Autodesk Fusion 360 part; units mm, degrees
(part 5 of 10)
  line L467 (-6.3, 22.99) -> (-5.3, 22.99)
  line L468 (-5.3, 20.36) -> (-5.3, 19.36)
  line L469 (-5.3, 19.36) -> (-6.3, 19.36)
  line L470 (-6.3, 19.36) -> (-6.3, 20.36)
  line L471 (-6.3, 20.36) -> (-5.3, 20.36)
  line L472 (-5.3, 17.73) -> (-5.3, 16.73)
  line L473 (-5.3, 16.73) -> (-6.3, 16.73)
  line L474 (-6.3, 16.73) -> (-6.3, 17.73)
  line L475 (-6.3, 17.73) -> (-5.3, 17.73)
  line L476 (-5.3, 15.1) -> (-5.3, 14.1)
  line L477 (-5.3, 14.1) -> (-6.3, 14.1)
  line L478 (-6.3, 14.1) -> (-6.3, 15.1)
  line L479 (-6.3, 15.1) -> (-5.3, 15.1)
  line L480 (-5.3, 12.47) -> (-5.3, 11.47)
  line L481 (-5.3, 11.47) -> (-6.3, 11.47)
  line L482 (-6.3, 11.47) -> (-6.3, 12.47)
  line L483 (-6.3, 12.47) -> (-5.3, 12.47)
  line L484 (-5.3, 9.84) -> (-5.3, 8.84)
  line L485 (-5.3, 8.84) -> (-6.3, 8.84)
  line L486 (-6.3, 8.84) -> (-6.3, 9.84)
  line L487 (-6.3, 9.84) -> (-5.3, 9.84)
  line L488 (-5.3, 7.21) -> (-5.3, 6.21)
  line L489 (-5.3, 6.21) -> (-6.3, 6.21)
  line L490 (-6.3, 6.21) -> (-6.3, 7.21)
  line L491 (-6.3, 7.21) -> (-5.3, 7.21)
  line L492 (-5.3, 4.58) -> (-5.3, 3.58)
  line L493 (-5.3, 3.58) -> (-6.3, 3.58)
  line L494 (-6.3, 3.58) -> (-6.3, 4.58)
  line L495 (-6.3, 4.58) -> (-5.3, 4.58)
  line L496 (-5.3, 1.95) -> (-5.3, 0.95)
  line L497 (-5.3, 0.95) -> (-6.3, 0.95)
  line L498 (-6.3, 0.95) -> (-6.3, 1.95)
  line L499 (-6.3, 1.95) -> (-5.3, 1.95)
  line L500 (-5.3, -0.68) -> (-5.3, -1.68)
  line L501 (-5.3, -1.68) -> (-6.3, -1.68)
  line L502 (-6.3, -1.68) -> (-6.3, -0.68)
  line L503 (-6.3, -0.68) -> (-5.3, -0.68)
  line L504 (-5.3, -3.31) -> (-5.3, -4.31)
  line L505 (-5.3, -4.31) -> (-6.3, -4.31)
  line L506 (-6.3, -4.31) -> (-6.3, -3.31)
  line L507 (-6.3, -3.31) -> (-5.3, -3.31)
  line L508 (-5.3, -5.94) -> (-5.3, -6.94)
  line L509 (-5.3, -6.94) -> (-6.3, -6.94)
  line L510 (-6.3, -6.94) -> (-6.3, -5.94)
  line L511 (-6.3, -5.94) -> (-5.3, -5.94)
  line L512 (-5.3, -8.57) -> (-5.3, -9.57)
  line L513 (-5.3, -9.57) -> (-6.3, -9.57)
  line L514 (-6.3, -9.57) -> (-6.3, -8.57)
  line L515 (-6.3, -8.57) -> (-5.3, -8.57)
  line L516 (-5.3, -11.2) -> (-5.3, -12.2)
  line L517 (-5.3, -12.2) -> (-6.3, -12.2)
  line L518 (-6.3, -12.2) -> (-6.3, -11.2)
  line L519 (-6.3, -11.2) -> (-5.3, -11.2)
  line L520 (-5.3, -13.83) -> (-5.3, -14.83)
  line L521 (-5.3, -14.83) -> (-6.3, -14.83)
  line L522 (-6.3, -14.83) -> (-6.3, -13.83)
  line L523 (-6.3, -13.83) -> (-5.3, -13.83)
  line L524 (-5.3, -16.46) -> (-5.3, -17.46)
  line L525 (-5.3, -17.46) -> (-6.3, -17.46)
  line L526 (-6.3, -17.46) -> (-6.3, -16.46)
  line L527 (-6.3, -16.46) -> (-5.3, -16.46)
  line L528 (-5.3, -19.09) -> (-5.3, -20.09)
  line L529 (-5.3, -20.09) -> (-6.3, -20.09)
  line L530 (-6.3, -20.09) -> (-6.3, -19.09)
  line L531 (-6.3, -19.09) -> (-5.3, -19.09)
  line L532 (-5.3, -21.72) -> (-5.3, -22.72)
  line L533 (-5.3, -22.72) -> (-6.3, -22.72)
  line L534 (-6.3, -22.72) -> (-6.3, -21.72)
  line L535 (-6.3, -21.72) -> (-5.3, -21.72)
  line L536 (-5.3, -24.35) -> (-5.3, -25.35)
  line L537 (-5.3, -25.35) -> (-6.3, -25.35)
  line L538 (-6.3, -25.35) -> (-6.3, -24.35)
  line L539 (-6.3, -24.35) -> (-5.3, -24.35)
  line L540 (-5.3, -26.98) -> (-5.3, -27.98)
  line L541 (-5.3, -27.98) -> (-6.3, -27.98)
  line L542 (-6.3, -27.98) -> (-6.3, -26.98)
  line L543 (-6.3, -26.98) -> (-5.3, -26.98)
  line L544 (-5.3, -29.61) -> (-5.3, -30.61)
  line L545 (-5.3, -30.61) -> (-6.3, -30.61)
  line L546 (-6.3, -30.61) -> (-6.3, -29.61)
  line L547 (-6.3, -29.61) -> (-5.3, -29.61)
  line L548 (-5.3, -32.24) -> (-5.3, -33.24)
  line L549 (-5.3, -33.24) -> (-6.3, -33.24)
  line L550 (-6.3, -33.24) -> (-6.3, -32.24)
  line L551 (-6.3, -32.24) -> (-5.3, -32.24)
  line L552 (-5.3, -34.87) -> (-5.3, -35.87)
  line L553 (-5.3, -35.87) -> (-6.3, -35.87)
  line L554 (-6.3, -35.87) -> (-6.3, -34.87)
  line L555 (-6.3, -34.87) -> (-5.3, -34.87)
  line L556 (-5.3, -37.5) -> (-5.3, -38.5)
  line L557 (-5.3, -38.5) -> (-6.3, -38.5)
  line L558 (-6.3, -38.5) -> (-6.3, -37.5)
  line L559 (-6.3, -37.5) -> (-5.3, -37.5)
  line L560 (-2.5, 38.77) -> (-2.5, 37.77)
  line L561 (-2.5, 37.77) -> (-3.5, 37.77)
  line L562 (-3.5, 37.77) -> (-3.5, 38.77)
  line L563 (-3.5, 38.77) -> (-2.5, 38.77)
  line L564 (-2.5, 36.14) -> (-2.5, 35.14)
  line L565 (-2.5, 35.14) -> (-3.5, 35.14)
  line L566 (-3.5, 35.14) -> (-3.5, 36.14)
  line L567 (-3.5, 36.14) -> (-2.5, 36.14)
  line L568 (-2.5, 33.51) -> (-2.5, 32.51)
  line L569 (-2.5, 32.51) -> (-3.5, 32.51)
  line L570 (-3.5, 32.51) -> (-3.5, 33.51)
  line L571 (-3.5, 33.51) -> (-2.5, 33.51)
  line L572 (-2.5, 30.88) -> (-2.5, 29.88)
  line L573 (-2.5, 29.88) -> (-3.5, 29.88)
  line L574 (-3.5, 29.88) -> (-3.5, 30.88)
  line L575 (-3.5, 30.88) -> (-2.5, 30.88)
  line L576 (-2.5, 28.25) -> (-2.5, 27.25)
  line L577 (-2.5, 27.25) -> (-3.5, 27.25)
  line L578 (-3.5, 27.25) -> (-3.5, 28.25)
  line L579 (-3.5, 28.25) -> (-2.5, 28.25)
  line L580 (-2.5, 25.62) -> (-2.5, 24.62)
  line L581 (-2.5, 24.62) -> (-3.5, 24.62)
  line L582 (-3.5, 24.62) -> (-3.5, 25.62)
  line L583 (-3.5, 25.62) -> (-2.5, 25.62)
  line L584 (-2.5, 22.99) -> (-2.5, 21.99)
  line L585 (-2.5, 21.99) -> (-3.5, 21.99)
  line L586 (-3.5, 21.99) -> (-3.5, 22.99)
  line L587 (-3.5, 22.99) -> (-2.5, 22.99)
  line L588 (-2.5, 20.36) -> (-2.5, 19.36)
  line L589 (-2.5, 19.36) -> (-3.5, 19.36)
  line L590 (-3.5, 19.36) -> (-3.5, 20.36)
  line L591 (-3.5, 20.36) -> (-2.5, 20.36)
  line L592 (-2.5, 17.73) -> (-2.5, 16.73)
  line L593 (-2.5, 16.73) -> (-3.5, 16.73)
  line L594 (-3.5, 16.73) -> (-3.5, 17.73)
  line L595 (-3.5, 17.73) -> (-2.5, 17.73)
  line L596 (-2.5, 15.1) -> (-2.5, 14.1)
  line L597 (-2.5, 14.1) -> (-3.5, 14.1)
  line L598 (-3.5, 14.1) -> (-3.5, 15.1)
  line L599 (-3.5, 15.1) -> (-2.5, 15.1)
  line L600 (-2.5, 12.47) -> (-2.5, 11.47)
  line L601 (-2.5, 11.47) -> (-3.5, 11.47)
  line L602 (-3.5, 11.47) -> (-3.5, 12.47)
  line L603 (-3.5, 12.47) -> (-2.5, 12.47)
  line L604 (-2.5, 9.84) -> (-2.5, 8.84)
  line L605 (-2.5, 8.84) -> (-3.5, 8.84)
  line L606 (-3.5, 8.84) -> (-3.5, 9.84)
  line L607 (-3.5, 9.84) -> (-2.5, 9.84)
  line L608 (-2.5, 7.21) -> (-2.5, 6.21)
  line L609 (-2.5, 6.21) -> (-3.5, 6.21)
  line L610 (-3.5, 6.21) -> (-3.5, 7.21)
  line L611 (-3.5, 7.21) -> (-2.5, 7.21)
  line L612 (-2.5, 4.58) -> (-2.5, 3.58)
  line L613 (-2.5, 3.58) -> (-3.5, 3.58)
  line L614 (-3.5, 3.58) -> (-3.5, 4.58)
  line L615 (-3.5, 4.58) -> (-2.5, 4.58)
  line L616 (-2.5, 1.95) -> (-2.5, 0.95)
  line L617 (-2.5, 0.95) -> (-3.5, 0.95)
  line L618 (-3.5, 0.95) -> (-3.5, 1.95)
  line L619 (-3.5, 1.95) -> (-2.5, 1.95)
  line L620 (-2.5, -0.68) -> (-2.5, -1.68)
  line L621 (-2.5, -1.68) -> (-3.5, -1.68)
  line L622 (-3.5, -1.68) -> (-3.5, -0.68)
  line L623 (-3.5, -0.68) -> (-2.5, -0.68)
  line L624 (-2.5, -3.31) -> (-2.5, -4.31)
  line L625 (-2.5, -4.31) -> (-3.5, -4.31)
  line L626 (-3.5, -4.31) -> (-3.5, -3.31)
  line L627 (-3.5, -3.31) -> (-2.5, -3.31)
  line L628 (-2.5, -5.94) -> (-2.5, -6.94)
  line L629 (-2.5, -6.94) -> (-3.5, -6.94)
  line L630 (-3.5, -6.94) -> (-3.5, -5.94)
  line L631 (-3.5, -5.94) -> (-2.5, -5.94)
  line L632 (-2.5, -8.57) -> (-2.5, -9.57)
  line L633 (-2.5, -9.57) -> (-3.5, -9.57)
  line L634 (-3.5, -9.57) -> (-3.5, -8.57)
  line L635 (-3.5, -8.57) -> (-2.5, -8.57)
  line L636 (-2.5, -11.2) -> (-2.5, -12.2)
  line L637 (-2.5, -12.2) -> (-3.5, -12.2)
  line L638 (-3.5, -12.2) -> (-3.5, -11.2)
  line L639 (-3.5, -11.2) -> (-2.5, -11.2)
  line L640 (-2.5, -13.83) -> (-2.5, -14.83)
  line L641 (-2.5, -14.83) -> (-3.5, -14.83)
  line L642 (-3.5, -14.83) -> (-3.5, -13.83)
  line L643 (-3.5, -13.83) -> (-2.5, -13.83)
  line L644 (-2.5, -16.46) -> (-2.5, -17.46)
  line L645 (-2.5, -17.46) -> (-3.5, -17.46)
  line L646 (-3.5, -17.46) -> (-3.5, -16.46)
  line L647 (-3.5, -16.46) -> (-2.5, -16.46)
  line L648 (-2.5, -19.09) -> (-2.5, -20.09)
  line L649 (-2.5, -20.09) -> (-3.5, -20.09)
  line L650 (-3.5, -20.09) -> (-3.5, -19.09)
  line L651 (-3.5, -19.09) -> (-2.5, -19.09)
  line L652 (-2.5, -21.72) -> (-2.5, -22.72)
  line L653 (-2.5, -22.72) -> (-3.5, -22.72)
  line L654 (-3.5, -22.72) -> (-3.5, -21.72)
  line L655 (-3.5, -21.72) -> (-2.5, -21.72)
  line L656 (-2.5, -24.35) -> (-2.5, -25.35)
  line L657 (-2.5, -25.35) -> (-3.5, -25.35)
  line L658 (-3.5, -25.35) -> (-3.5, -24.35)
  line L659 (-3.5, -24.35) -> (-2.5, -24.35)
  line L660 (-2.5, -26.98) -> (-2.5, -27.98)
  line L661 (-2.5, -27.98) -> (-3.5, -27.98)
  line L662 (-3.5, -27.98) -> (-3.5, -26.98)
  line L663 (-3.5, -26.98) -> (-2.5, -26.98)
  line L664 (-2.5, -29.61) -> (-2.5, -30.61)
  line L665 (-2.5, -30.61) -> (-3.5, -30.61)
  line L666 (-3.5, -30.61) -> (-3.5, -29.61)
  line L667 (-3.5, -29.61) -> (-2.5, -29.61)
  line L668 (-2.5, -32.24) -> (-2.5, -33.24)
  line L669 (-2.5, -33.24) -> (-3.5, -33.24)
  line L670 (-3.5, -33.24) -> (-3.5, -32.24)
  line L671 (-3.5, -32.24) -> (-2.5, -32.24)
  line L672 (-2.5, -34.87) -> (-2.5, -35.87)
  line L673 (-2.5, -35.87) -> (-3.5, -35.87)
  line L674 (-3.5, -35.87) -> (-3.5, -34.87)
  line L675 (-3.5, -34.87) -> (-2.5, -34.87)
  line L676 (-2.5, -37.5) -> (-2.5, -38.5)
  line L677 (-2.5, -38.5) -> (-3.5, -38.5)
  line L678 (-3.5, -38.5) -> (-3.5, -37.5)
  line L679 (-3.5, -37.5) -> (-2.5, -37.5)
  line L680 (-1, -40.5) -> (-1, 40.5)
  line L681 (-1, 40.5) -> (-26.5, 40.5)
  line L682 (-26.5, 40.5) -> (-26.5, -40.5)
  line L683 (-26.5, -40.5) -> (-1, -40.5)
  line L684 (-23.998, -5.06) -> (-22.998, -5.06)
  line L685 (-22.998, -5.06) -> (-22.998, -6.06)
  line L686 (-22.998, -6.06) -> (-23.998, -6.06)
  line L687 (-23.998, -6.06) -> (-23.998, -5.06)
  line L688 (-23.998, -5.06) -> (-22.998, -6.06) construction
  line L689 (-22.998, -5.06) -> (-23.998, -6.06) construction
  point P0 (-23.498, -5.56)
  dimension "d188" = 1
  dimension "d189" = 1
  dimension "d190" = 3.7
  constraint horizontal L684
  constraint perpendicular L684 L685
  constraint parallel L684 L686
  constraint parallel L685 L687
  constraint coincident L688 P0
  constraint coincident L689 P0
  measures "d188" distance of L684.start L686.end
  measures "d189" distance of L685.end L686.end
  measures "d190" distance of L7 L686
extrude "Extrude31" cut sketch "Sketch31" against normal blind 1 contours L684 L685 L686 L687 bodies 1
pattern_linear "R-Pattern9" count 2 spacing 3 along (-1, 0, 0) count 5 spacing 2.63 along (0, -1, 0) of "Extrude31"
sketch "Sketch32" plane through (0, 0, 9) normal (0, 0, 1) x (-1, 0, 0)
  line L0 (-19.998, 5.46) -> (-19.998, 4.46)
  line L1 (-19.998, 4.46) -> (-20.998, 4.46)
  line L2 (-20.998, 4.46) -> (-20.998, 5.46)
  line L3 (-20.998, 5.46) -> (-19.998, 5.46)
  line L4 (-22.998, 5.46) -> (-22.998, 4.46)
  line L5 (-22.998, 4.46) -> (-23.998, 4.46)
  line L6 (-23.998, 4.46) -> (-23.998, 5.46)
  line L7 (-23.998, 5.46) -> (-22.998, 5.46)
  line L8 (-19.998, 2.83) -> (-19.998, 1.83)
  line L9 (-19.998, 1.83) -> (-20.998, 1.83)
  line L10 (-20.998, 1.83) -> (-20.998, 2.83)
  line L11 (-20.998, 2.83) -> (-19.998, 2.83)
  line L12 (-22.998, 2.83) -> (-22.998, 1.83)
  line L13 (-22.998, 1.83) -> (-23.998, 1.83)
  line L14 (-23.998, 1.83) -> (-23.998, 2.83)
  line L15 (-23.998, 2.83) -> (-22.998, 2.83)
  line L16 (-19.998, 0.2) -> (-19.998, -0.8)
  line L17 (-19.998, -0.8) -> (-20.998, -0.8)
  line L18 (-20.998, -0.8) -> (-20.998, 0.2)
  line L19 (-20.998, 0.2) -> (-19.998, 0.2)
  line L20 (-22.998, 0.2) -> (-22.998, -0.8)
  line L21 (-22.998, -0.8) -> (-23.998, -0.8)
  line L22 (-23.998, -0.8) -> (-23.998, 0.2)
  line L23 (-23.998, 0.2) -> (-22.998, 0.2)
  line L24 (-19.998, -2.43) -> (-19.998, -3.43)
  line L25 (-19.998, -3.43) -> (-20.998, -3.43)
  line L26 (-20.998, -3.43) -> (-20.998, -2.43)
  line L27 (-20.998, -2.43) -> (-19.998, -2.43)
  line L28 (-22.998, -2.43) -> (-22.998, -3.43)
  line L29 (-22.998, -3.43) -> (-23.998, -3.43)
  line L30 (-23.998, -3.43) -> (-23.998, -2.43)
  line L31 (-23.998, -2.43) -> (-22.998, -2.43)
  line L32 (-19.998, -5.06) -> (-19.998, -6.06)
  line L33 (-19.998, -6.06) -> (-20.998, -6.06)
  line L34 (-20.998, -6.06) -> (-20.998, -5.06)
  line L35 (-20.998, -5.06) -> (-19.998, -5.06)
  line L36 (-22.998, -5.06) -> (-22.998, -6.06)
  line L37 (-22.998, -6.06) -> (-23.998, -6.06)
  line L38 (-23.998, -6.06) -> (-23.998, -5.06)
  line L39 (-23.998, -5.06) -> (-22.998, -5.06)
  line L40 (-20, -9.76) -> (-20, -10.76)
  line L41 (-20, -10.76) -> (-21, -10.76)
  line L42 (-21, -10.76) -> (-21, -9.76)
  line L43 (-21, -9.76) -> (-20, -9.76)
  line L44 (-23, -9.76) -> (-23, -10.76)
  line L45 (-23, -10.76) -> (-24, -10.76)
  line L46 (-24, -10.76) -> (-24, -9.76)
  line L47 (-24, -9.76) -> (-23, -9.76)
  line L48 (-20, -12.39) -> (-20, -13.39)
  line L49 (-20, -13.39) -> (-21, -13.39)
  line L50 (-21, -13.39) -> (-21, -12.39)
  line L51 (-21, -12.39) -> (-20, -12.39)
  line L52 (-23, -12.39) -> (-23, -13.39)
  line L53 (-23, -13.39) -> (-24, -13.39)
  line L54 (-24, -13.39) -> (-24, -12.39)
  line L55 (-24, -12.39) -> (-23, -12.39)
  line L56 (-20, -15.02) -> (-20, -16.02)
  line L57 (-20, -16.02) -> (-21, -16.02)
  line L58 (-21, -16.02) -> (-21, -15.02)
  line L59 (-21, -15.02) -> (-20, -15.02)
  line L60 (-23, -15.02) -> (-23, -16.02)
  line L61 (-23, -16.02) -> (-24, -16.02)
  line L62 (-24, -16.02) -> (-24, -15.02)
  line L63 (-24, -15.02) -> (-23, -15.02)
  line L64 (-20, -17.65) -> (-20, -18.65)
  line L65 (-20, -18.65) -> (-21, -18.65)
  line L66 (-21, -18.65) -> (-21, -17.65)
  line L67 (-21, -17.65) -> (-20, -17.65)
  line L68 (-23, -17.65) -> (-23, -18.65)
  line L69 (-23, -18.65) -> (-24, -18.65)
  line L70 (-24, -18.65) -> (-24, -17.65)
  line L71 (-24, -17.65) -> (-23, -17.65)
  line L72 (-20, -20.28) -> (-20, -21.28)
  line L73 (-20, -21.28) -> (-21, -21.28)
  line L74 (-21, -21.28) -> (-21, -20.28)
  line L75 (-21, -20.28) -> (-20, -20.28)
  line L76 (-23, -20.28) -> (-23, -21.28)
  line L77 (-23, -21.28) -> (-24, -21.28)
  line L78 (-24, -21.28) -> (-24, -20.28)
  line L79 (-24, -20.28) -> (-23, -20.28)
  line L80 (-20, -24.98) -> (-20, -25.98)
  line L81 (-20, -25.98) -> (-21, -25.98)
  line L82 (-21, -25.98) -> (-21, -24.98)
  line L83 (-21, -24.98) -> (-20, -24.98)
  line L84 (-23, -24.98) -> (-23, -25.98)
  line L85 (-23, -25.98) -> (-24, -25.98)
  line L86 (-24, -25.98) -> (-24, -24.98)
  line L87 (-24, -24.98) -> (-23, -24.98)
  line L88 (-20, -27.61) -> (-20, -28.61)
  line L89 (-20, -28.61) -> (-21, -28.61)
  line L90 (-21, -28.61) -> (-21, -27.61)
  line L91 (-21, -27.61) -> (-20, -27.61)
  line L92 (-23, -27.61) -> (-23, -28.61)
  line L93 (-23, -28.61) -> (-24, -28.61)
  line L94 (-24, -28.61) -> (-24, -27.61)
  line L95 (-24, -27.61) -> (-23, -27.61)
  line L96 (-20, -30.24) -> (-20, -31.24)
  line L97 (-20, -31.24) -> (-21, -31.24)
  line L98 (-21, -31.24) -> (-21, -30.24)
  line L99 (-21, -30.24) -> (-20, -30.24)
  line L100 (-23, -30.24) -> (-23, -31.24)
  line L101 (-23, -31.24) -> (-24, -31.24)
  line L102 (-24, -31.24) -> (-24, -30.24)
  line L103 (-24, -30.24) -> (-23, -30.24)
  line L104 (-20, -32.87) -> (-20, -33.87)
  line L105 (-20, -33.87) -> (-21, -33.87)
  line L106 (-21, -33.87) -> (-21, -32.87)
  line L107 (-21, -32.87) -> (-20, -32.87)
  line L108 (-23, -32.87) -> (-23, -33.87)
  line L109 (-23, -33.87) -> (-24, -33.87)
  line L110 (-24, -33.87) -> (-24, -32.87)
  line L111 (-24, -32.87) -> (-23, -32.87)
  line L112 (-20, -35.5) -> (-20, -36.5)
  line L113 (-20, -36.5) -> (-21, -36.5)
  line L114 (-21, -36.5) -> (-21, -35.5)
  line L115 (-21, -35.5) -> (-20, -35.5)
  line L116 (-23, -35.5) -> (-23, -36.5)
  line L117 (-23, -36.5) -> (-24, -36.5)
  line L118 (-24, -36.5) -> (-24, -35.5)
  line L119 (-24, -35.5) -> (-23, -35.5)
  line L120 (-13.7, 38.77) -> (-13.7, 37.77)
  line L121 (-13.7, 37.77) -> (-14.7, 37.77)
  line L122 (-14.7, 37.77) -> (-14.7, 38.77)
  line L123 (-14.7, 38.77) -> (-13.7, 38.77)
  line L124 (-13.7, 36.14) -> (-13.7, 35.14)
  line L125 (-13.7, 35.14) -> (-14.7, 35.14)
  line L126 (-14.7, 35.14) -> (-14.7, 36.14)
  line L127 (-14.7, 36.14) -> (-13.7, 36.14)
  line L128 (-13.7, 33.51) -> (-13.7, 32.51)
  line L129 (-13.7, 32.51) -> (-14.7, 32.51)
  line L130 (-14.7, 32.51) -> (-14.7, 33.51)
  line L131 (-14.7, 33.51) -> (-13.7, 33.51)
  line L132 (-13.7, 30.88) -> (-13.7, 29.88)
  line L133 (-13.7, 29.88) -> (-14.7, 29.88)
  line L134 (-14.7, 29.88) -> (-14.7, 30.88)
  line L135 (-14.7, 30.88) -> (-13.7, 30.88)
  line L136 (-13.7, 28.25) -> (-13.7, 27.25)
  line L137 (-13.7, 27.25) -> (-14.7, 27.25)
  line L138 (-14.7, 27.25) -> (-14.7, 28.25)
  line L139 (-14.7, 28.25) -> (-13.7, 28.25)
  line L140 (-13.7, 25.62) -> (-13.7, 24.62)
  line L141 (-13.7, 24.62) -> (-14.7, 24.62)
  line L142 (-14.7, 24.62) -> (-14.7, 25.62)
  line L143 (-14.7, 25.62) -> (-13.7, 25.62)
  line L144 (-13.7, 22.99) -> (-13.7, 21.99)
  line L145 (-13.7, 21.99) -> (-14.7, 21.99)
  line L146 (-14.7, 21.99) -> (-14.7, 22.99)
  line L147 (-14.7, 22.99) -> (-13.7, 22.99)
  line L148 (-13.7, 20.36) -> (-13.7, 19.36)
  line L149 (-13.7, 19.36) -> (-14.7, 19.36)
  line L150 (-14.7, 19.36) -> (-14.7, 20.36)
  line L151 (-14.7, 20.36) -> (-13.7, 20.36)
  line L152 (-13.7, 17.73) -> (-13.7, 16.73)
  line L153 (-13.7, 16.73) -> (-14.7, 16.73)
  line L154 (-14.7, 16.73) -> (-14.7, 17.73)
  line L155 (-14.7, 17.73) -> (-13.7, 17.73)
  line L156 (-13.7, 15.1) -> (-13.7, 14.1)
  line L157 (-13.7, 14.1) -> (-14.7, 14.1)
  line L158 (-14.7, 14.1) -> (-14.7, 15.1)
  line L159 (-14.7, 15.1) -> (-13.7, 15.1)
  line L160 (-13.7, 12.47) -> (-13.7, 11.47)
  line L161 (-13.7, 11.47) -> (-14.7, 11.47)
  line L162 (-14.7, 11.47) -> (-14.7, 12.47)
  line L163 (-14.7, 12.47) -> (-13.7, 12.47)
  line L164 (-13.7, 9.84) -> (-13.7, 8.84)
  line L165 (-13.7, 8.84) -> (-14.7, 8.84)
  line L166 (-14.7, 8.84) -> (-14.7, 9.84)
  line L167 (-14.7, 9.84) -> (-13.7, 9.84)
  line L168 (-13.7, 7.21) -> (-13.7, 6.21)
  line L169 (-13.7, 6.21) -> (-14.7, 6.21)
  line L170 (-14.7, 6.21) -> (-14.7, 7.21)
  line L171 (-14.7, 7.21) -> (-13.7, 7.21)
  line L172 (-13.7, 4.58) -> (-13.7, 3.58)
  line L173 (-13.7, 3.58) -> (-14.7, 3.58)
  line L174 (-14.7, 3.58) -> (-14.7, 4.58)
  line L175 (-14.7, 4.58) -> (-13.7, 4.58)
  line L176 (-13.7, 1.95) -> (-13.7, 0.95)
  line L177 (-13.7, 0.95) -> (-14.7, 0.95)
  line L178 (-14.7, 0.95) -> (-14.7, 1.95)
  line L179 (-14.7, 1.95) -> (-13.7, 1.95)
  line L180 (-13.7, -0.68) -> (-13.7, -1.68)
  line L181 (-13.7, -1.68) -> (-14.7, -1.68)
  line L182 (-14.7, -1.68) -> (-14.7, -0.68)
  line L183 (-14.7, -0.68) -> (-13.7, -0.68)
  line L184 (-13.7, -3.31) -> (-13.7, -4.31)
  line L185 (-13.7, -4.31) -> (-14.7, -4.31)
  line L186 (-14.7, -4.31) -> (-14.7, -3.31)
  line L187 (-14.7, -3.31) -> (-13.7, -3.31)
  line L188 (-13.7, -5.94) -> (-13.7, -6.94)
  line L189 (-13.7, -6.94) -> (-14.7, -6.94)
  line L190 (-14.7, -6.94) -> (-14.7, -5.94)
  line L191 (-14.7, -5.94) -> (-13.7, -5.94)
  line L192 (-13.7, -8.57) -> (-13.7, -9.57)
  line L193 (-13.7, -9.57) -> (-14.7, -9.57)
  line L194 (-14.7, -9.57) -> (-14.7, -8.57)
  line L195 (-14.7, -8.57) -> (-13.7, -8.57)
  line L196 (-13.7, -11.2) -> (-13.7, -12.2)
  line L197 (-13.7, -12.2) -> (-14.7, -12.2)
  line L198 (-14.7, -12.2) -> (-14.7, -11.2)
  line L199 (-14.7, -11.2) -> (-13.7, -11.2)
  line L200 (-13.7, -13.83) -> (-13.7, -14.83)
  line L201 (-13.7, -14.83) -> (-14.7, -14.83)
  line L202 (-14.7, -14.83) -> (-14.7, -13.83)
  line L203 (-14.7, -13.83) -> (-13.7, -13.83)
  line L204 (-13.7, -16.46) -> (-13.7, -17.46)
  line L205 (-13.7, -17.46) -> (-14.7, -17.46)
  line L206 (-14.7, -17.46) -> (-14.7, -16.46)
  line L207 (-14.7, -16.46) -> (-13.7, -16.46)
  line L208 (-13.7, -19.09) -> (-13.7, -20.09)
  line L209 (-13.7, -20.09) -> (-14.7, -20.09)
  line L210 (-14.7, -20.09) -> (-14.7, -19.09)
  line L211 (-14.7, -19.09) -> (-13.7, -19.09)
  line L212 (-13.7, -21.72) -> (-13.7, -22.72)
  line L213 (-13.7, -22.72) -> (-14.7, -22.72)
  line L214 (-14.7, -22.72) -> (-14.7, -21.72)
  line L215 (-14.7, -21.72) -> (-13.7, -21.72)
  line L216 (-13.7, -24.35) -> (-13.7, -25.35)
  line L217 (-13.7, -25.35) -> (-14.7, -25.35)
  line L218 (-14.7, -25.35) -> (-14.7, -24.35)
  line L219 (-14.7, -24.35) -> (-13.7, -24.35)
  line L220 (-13.7, -26.98) -> (-13.7, -27.98)
  line L221 (-13.7, -27.98) -> (-14.7, -27.98)
  line L222 (-14.7, -27.98) -> (-14.7, -26.98)
  line L223 (-14.7, -26.98) -> (-13.7, -26.98)
  line L224 (-13.7, -29.61) -> (-13.7, -30.61)
  line L225 (-13.7, -30.61) -> (-14.7, -30.61)
  line L226 (-14.7, -30.61) -> (-14.7, -29.61)
  line L227 (-14.7, -29.61) -> (-13.7, -29.61)
  line L228 (-13.7, -32.24) -> (-13.7, -33.24)
  line L229 (-13.7, -33.24) -> (-14.7, -33.24)
  line L230 (-14.7, -33.24) -> (-14.7, -32.24)
  line L231 (-14.7, -32.24) -> (-13.7, -32.24)
  line L232 (-13.7, -34.87) -> (-13.7, -35.87)
  line L233 (-13.7, -35.87) -> (-14.7, -35.87)
  line L234 (-14.7, -35.87) -> (-14.7, -34.87)
  line L235 (-14.7, -34.87) -> (-13.7, -34.87)
  line L236 (-13.7, -37.5) -> (-13.7, -38.5)
  line L237 (-13.7, -38.5) -> (-14.7, -38.5)
  line L238 (-14.7, -38.5) -> (-14.7, -37.5)
  line L239 (-14.7, -37.5) -> (-13.7, -37.5)
  line L240 (-10.9, 38.77) -> (-10.9, 37.77)
  line L241 (-10.9, 37.77) -> (-11.9, 37.77)
  line L242 (-11.9, 37.77) -> (-11.9, 38.77)
  line L243 (-11.9, 38.77) -> (-10.9, 38.77)
  line L244 (-10.9, 36.14) -> (-10.9, 35.14)
  line L245 (-10.9, 35.14) -> (-11.9, 35.14)
  line L246 (-11.9, 35.14) -> (-11.9, 36.14)
  line L247 (-11.9, 36.14) -> (-10.9, 36.14)
  line L248 (-10.9, 33.51) -> (-10.9, 32.51)
  line L249 (-10.9, 32.51) -> (-11.9, 32.51)
  line L250 (-11.9, 32.51) -> (-11.9, 33.51)
  line L251 (-11.9, 33.51) -> (-10.9, 33.51)
  line L252 (-10.9, 30.88) -> (-10.9, 29.88)
  line L253 (-10.9, 29.88) -> (-11.9, 29.88)
  line L254 (-11.9, 29.88) -> (-11.9, 30.88)
  line L255 (-11.9, 30.88) -> (-10.9, 30.88)
  line L256 (-10.9, 28.25) -> (-10.9, 27.25)
  line L257 (-10.9, 27.25) -> (-11.9, 27.25)
  line L258 (-11.9, 27.25) -> (-11.9, 28.25)
  line L259 (-11.9, 28.25) -> (-10.9, 28.25)
  line L260 (-10.9, 25.62) -> (-10.9, 24.62)
  line L261 (-10.9, 24.62) -> (-11.9, 24.62)
  line L262 (-11.9, 24.62) -> (-11.9, 25.62)
  line L263 (-11.9, 25.62) -> (-10.9, 25.62)
  line L264 (-10.9, 22.99) -> (-10.9, 21.99)
  line L265 (-10.9, 21.99) -> (-11.9, 21.99)
  line L266 (-11.9, 21.99) -> (-11.9, 22.99)
  line L267 (-11.9, 22.99) -> (-10.9, 22.99)
  line L268 (-10.9, 20.36) -> (-10.9, 19.36)
  line L269 (-10.9, 19.36) -> (-11.9, 19.36)
  line L270 (-11.9, 19.36) -> (-11.9, 20.36)
  line L271 (-11.9, 20.36) -> (-10.9, 20.36)
  line L272 (-10.9, 17.73) -> (-10.9, 16.73)
  line L273 (-10.9, 16.73) -> (-11.9, 16.73)
  line L274 (-11.9, 16.73) -> (-11.9, 17.73)
  line L275 (-11.9, 17.73) -> (-10.9, 17.73)
  line L276 (-10.9, 15.1) -> (-10.9, 14.1)
  line L277 (-10.9, 14.1) -> (-11.9, 14.1)
  line L278 (-11.9, 14.1) -> (-11.9, 15.1)
  line L279 (-11.9, 15.1) -> (-10.9, 15.1)
  line L280 (-10.9, 12.47) -> (-10.9, 11.47)
  line L281 (-10.9, 11.47) -> (-11.9, 11.47)
  line L282 (-11.9, 11.47) -> (-11.9, 12.47)
  line L283 (-11.9, 12.47) -> (-10.9, 12.47)
  line L284 (-10.9, 9.84) -> (-10.9, 8.84)
  line L285 (-10.9, 8.84) -> (-11.9, 8.84)
  line L286 (-11.9, 8.84) -> (-11.9, 9.84)
  line L287 (-11.9, 9.84) -> (-10.9, 9.84)
  line L288 (-10.9, 7.21) -> (-10.9, 6.21)
  line L289 (-10.9, 6.21) -> (-11.9, 6.21)
  line L290 (-11.9, 6.21) -> (-11.9, 7.21)
  line L291 (-11.9, 7.21) -> (-10.9, 7.21)
  line L292 (-10.9, 4.58) -> (-10.9, 3.58)
  line L293 (-10.9, 3.58) -> (-11.9, 3.58)
  line L294 (-11.9, 3.58) -> (-11.9, 4.58)
  line L295 (-11.9, 4.58) -> (-10.9, 4.58)
  line L296 (-10.9, 1.95) -> (-10.9, 0.95)
  line L297 (-10.9, 0.95) -> (-11.9, 0.95)
  line L298 (-11.9, 0.95) -> (-11.9, 1.95)
  line L299 (-11.9, 1.95) -> (-10.9, 1.95)
  line L300 (-10.9, -0.68) -> (-10.9, -1.68)
  line L301 (-10.9, -1.68) -> (-11.9, -1.68)
  line L302 (-11.9, -1.68) -> (-11.9, -0.68)
  line L303 (-11.9, -0.68) -> (-10.9, -0.68)
  line L304 (-10.9, -3.31) -> (-10.9, -4.31)
  line L305 (-10.9, -4.31) -> (-11.9, -4.31)
  line L306 (-11.9, -4.31) -> (-11.9, -3.31)
  line L307 (-11.9, -3.31) -> (-10.9, -3.31)
  line L308 (-10.9, -5.94) -> (-10.9, -6.94)
  line L309 (-10.9, -6.94) -> (-11.9, -6.94)
  line L310 (-11.9, -6.94) -> (-11.9, -5.94)
  line L311 (-11.9, -5.94) -> (-10.9, -5.94)
  line L312 (-10.9, -8.57) -> (-10.9, -9.57)
  line L313 (-10.9, -9.57) -> (-11.9, -9.57)
  line L314 (-11.9, -9.57) -> (-11.9, -8.57)
  line L315 (-11.9, -8.57) -> (-10.9, -8.57)
  line L316 (-10.9, -11.2) -> (-10.9, -12.2)
  line L317 (-10.9, -12.2) -> (-11.9, -12.2)
  line L318 (-11.9, -12.2) -> (-11.9, -11.2)
  line L319 (-11.9, -11.2) -> (-10.9, -11.2)
  line L320 (-10.9, -13.83) -> (-10.9, -14.83)
  line L321 (-10.9, -14.83) -> (-11.9, -14.83)
  line L322 (-11.9, -14.83) -> (-11.9, -13.83)
  line L323 (-11.9, -13.83) -> (-10.9, -13.83)
  line L324 (-10.9, -16.46) -> (-10.9, -17.46)
  line L325 (-10.9, -17.46) -> (-11.9, -17.46)
  line L326 (-11.9, -17.46) -> (-11.9, -16.46)
  line L327 (-11.9, -16.46) -> (-10.9, -16.46)
  line L328 (-10.9, -19.09) -> (-10.9, -20.09)
  line L329 (-10.9, -20.09) -> (-11.9, -20.09)
  line L330 (-11.9, -20.09) -> (-11.9, -19.09)
  line L331 (-11.9, -19.09) -> (-10.9, -19.09)
  line L332 (-10.9, -21.72) -> (-10.9, -22.72)
  line L333 (-10.9, -22.72) -> (-11.9, -22.72)
  line L334 (-11.9, -22.72) -> (-11.9, -21.72)
  line L335 (-11.9, -21.72) -> (-10.9, -21.72)
  line L336 (-10.9, -24.35) -> (-10.9, -25.35)
  line L337 (-10.9, -25.35) -> (-11.9, -25.35)
  line L338 (-11.9, -25.35) -> (-11.9, -24.35)
  line L339 (-11.9, -24.35) -> (-10.9, -24.35)
  line L340 (-10.9, -26.98) -> (-10.9, -27.98)
  line L341 (-10.9, -27.98) -> (-11.9, -27.98)
  line L342 (-11.9, -27.98) -> (-11.9, -26.98)
  line L343 (-11.9, -26.98) -> (-10.9, -26.98)
  line L344 (-10.9, -29.61) -> (-10.9, -30.61)
  line L345 (-10.9, -30.61) -> (-11.9, -30.61)
  line L346 (-11.9, -30.61) -> (-11.9, -29.61)
  line L347 (-11.9, -29.61) -> (-10.9, -29.61)
  line L348 (-10.9, -32.24) -> (-10.9, -33.24)
  line L349 (-10.9, -33.24) -> (-11.9, -33.24)
  line L350 (-11.9, -33.24) -> (-11.9, -32.24)
  line L351 (-11.9, -32.24) -> (-10.9, -32.24)
  line L352 (-10.9, -34.87) -> (-10.9, -35.87)
  line L353 (-10.9, -35.87) -> (-11.9, -35.87)
  line L354 (-11.9, -35.87) -> (-11.9, -34.87)
  line L355 (-11.9, -34.87) -> (-10.9, -34.87)
  line L356 (-10.9, -37.5) -> (-10.9, -38.5)
  line L357 (-10.9, -38.5) -> (-11.9, -38.5)
  line L358 (-11.9, -38.5) -> (-11.9, -37.5)
  line L359 (-11.9, -37.5) -> (-10.9, -37.5)
  line L360 (-8.1, 38.77) -> (-8.1, 37.77)
  line L361 (-8.1, 37.77) -> (-9.1, 37.77)
  line L362 (-9.1, 37.77) -> (-9.1, 38.77)
  line L363 (-9.1, 38.77) -> (-8.1, 38.77)
  line L364 (-8.1, 36.14) -> (-8.1, 35.14)
  line L365 (-8.1, 35.14) -> (-9.1, 35.14)
  line L366 (-9.1, 35.14) -> (-9.1, 36.14)
  line L367 (-9.1, 36.14) -> (-8.1, 36.14)
  line L368 (-8.1, 33.51) -> (-8.1, 32.51)
  line L369 (-8.1, 32.51) -> (-9.1, 32.51)
  line L370 (-9.1, 32.51) -> (-9.1, 33.51)
  line L371 (-9.1, 33.51) -> (-8.1, 33.51)
  line L372 (-8.1, 30.88) -> (-8.1, 29.88)
  line L373 (-8.1, 29.88) -> (-9.1, 29.88)
  line L374 (-9.1, 29.88) -> (-9.1, 30.88)
  line L375 (-9.1, 30.88) -> (-8.1, 30.88)
  line L376 (-8.1, 28.25) -> (-8.1, 27.25)
  line L377 (-8.1, 27.25) -> (-9.1, 27.25)
  line L378 (-9.1, 27.25) -> (-9.1, 28.25)
  line L379 (-9.1, 28.25) -> (-8.1, 28.25)
  line L380 (-8.1, 25.62) -> (-8.1, 24.62)
  line L381 (-8.1, 24.62) -> (-9.1, 24.62)
  line L382 (-9.1, 24.62) -> (-9.1, 25.62)
  line L383 (-9.1, 25.62) -> (-8.1, 25.62)
  line L384 (-8.1, 22.99) -> (-8.1, 21.99)
  line L385 (-8.1, 21.99) -> (-9.1, 21.99)
  line L386 (-9.1, 21.99) -> (-9.1, 22.99)
  line L387 (-9.1, 22.99) -> (-8.1, 22.99)
  line L388 (-8.1, 20.36) -> (-8.1, 19.36)
  line L389 (-8.1, 19.36) -> (-9.1, 19.36)
  line L390 (-9.1, 19.36) -> (-9.1, 20.36)
  line L391 (-9.1, 20.36) -> (-8.1, 20.36)
  line L392 (-8.1, 17.73) -> (-8.1, 16.73)
  line L393 (-8.1, 16.73) -> (-9.1, 16.73)
  line L394 (-9.1, 16.73) -> (-9.1, 17.73)
  line L395 (-9.1, 17.73) -> (-8.1, 17.73)
  line L396 (-8.1, 15.1) -> (-8.1, 14.1)
  line L397 (-8.1, 14.1) -> (-9.1, 14.1)
  line L398 (-9.1, 14.1) -> (-9.1, 15.1)
  line L399 (-9.1, 15.1) -> (-8.1, 15.1)
  line L400 (-8.1, 12.47) -> (-8.1, 11.47)
  line L401 (-8.1, 11.47) -> (-9.1, 11.47)
  line L402 (-9.1, 11.47) -> (-9.1, 12.47)
  line L403 (-9.1, 12.47) -> (-8.1, 12.47)
  line L404 (-8.1, 9.84) -> (-8.1, 8.84)
  line L405 (-8.1, 8.84) -> (-9.1, 8.84)
  line L406 (-9.1, 8.84) -> (-9.1, 9.84)
  line L407 (-9.1, 9.84) -> (-8.1, 9.84)
  line L408 (-8.1, 7.21) -> (-8.1, 6.21)
  line L409 (-8.1, 6.21) -> (-9.1, 6.21)
  line L410 (-9.1, 6.21) -> (-9.1, 7.21)
  line L411 (-9.1, 7.21) -> (-8.1, 7.21)
  line L412 (-8.1, 4.58) -> (-8.1, 3.58)
  line L413 (-8.1, 3.58) -> (-9.1, 3.58)
  line L414 (-9.1, 3.58) -> (-9.1, 4.58)
  line L415 (-9.1, 4.58) -> (-8.1, 4.58)
  line L416 (-8.1, 1.95) -> (-8.1, 0.95)
  line L417 (-8.1, 0.95) -> (-9.1, 0.95)
  line L418 (-9.1, 0.95) -> (-9.1, 1.95)
  line L419 (-9.1, 1.95) -> (-8.1, 1.95)
  line L420 (-8.1, -0.68) -> (-8.1, -1.68)
  line L421 (-8.1, -1.68) -> (-9.1, -1.68)
  line L422 (-9.1, -1.68) -> (-9.1, -0.68)
  line L423 (-9.1, -0.68) -> (-8.1, -0.68)
  line L424 (-8.1, -3.31) -> (-8.1, -4.31)
  line L425 (-8.1, -4.31) -> (-9.1, -4.31)
  line L426 (-9.1, -4.31) -> (-9.1, -3.31)
  line L427 (-9.1, -3.31) -> (-8.1, -3.31)
  line L428 (-8.1, -5.94) -> (-8.1, -6.94)
  line L429 (-8.1, -6.94) -> (-9.1, -6.94)
  line L430 (-9.1, -6.94) -> (-9.1, -5.94)
  line L431 (-9.1, -5.94) -> (-8.1, -5.94)
  line L432 (-8.1, -8.57) -> (-8.1, -9.57)
  line L433 (-8.1, -9.57) -> (-9.1, -9.57)
  line L434 (-9.1, -9.57) -> (-9.1, -8.57)
  line L435 (-9.1, -8.57) -> (-8.1, -8.57)
  line L436 (-8.1, -11.2) -> (-8.1, -12.2)
  line L437 (-8.1, -12.2) -> (-9.1, -12.2)
  line L438 (-9.1, -12.2) -> (-9.1, -11.2)
  line L439 (-9.1, -11.2) -> (-8.1, -11.2)
  line L440 (-8.1, -13.83) -> (-8.1, -14.83)
  line L441 (-8.1, -14.83) -> (-9.1, -14.83)
  line L442 (-9.1, -14.83) -> (-9.1, -13.83)
  line L443 (-9.1, -13.83) -> (-8.1, -13.83)
  line L444 (-8.1, -16.46) -> (-8.1, -17.46)
  line L445 (-8.1, -17.46) -> (-9.1, -17.46)
  line L446 (-9.1, -17.46) -> (-9.1, -16.46)
  line L447 (-9.1, -16.46) -> (-8.1, -16.46)
  line L448 (-8.1, -19.09) -> (-8.1, -20.09)
  line L449 (-8.1, -20.09) -> (-9.1, -20.09)
  line L450 (-9.1, -20.09) -> (-9.1, -19.09)
  line L451 (-9.1, -19.09) -> (-8.1, -19.09)
  line L452 (-8.1, -21.72) -> (-8.1, -22.72)
  line L453 (-8.1, -22.72) -> (-9.1, -22.72)
  line L454 (-9.1, -22.72) -> (-9.1, -21.72)
  line L455 (-9.1, -21.72) -> (-8.1, -21.72)
  line L456 (-8.1, -24.35) -> (-8.1, -25.35)
  line L457 (-8.1, -25.35) -> (-9.1, -25.35)
  line L458 (-9.1, -25.35) -> (-9.1, -24.35)
  line L459 (-9.1, -24.35) -> (-8.1, -24.35)
  line L460 (-8.1, -26.98) -> (-8.1, -27.98)
  line L461 (-8.1, -27.98) -> (-9.1, -27.98)
  line L462 (-9.1, -27.98) -> (-9.1, -26.98)
  line L463 (-9.1, -26.98) -> (-8.1, -26.98)
  line L464 (-8.1, -29.61) -> (-8.1, -30.61)
  line L465 (-8.1, -30.61) -> (-9.1, -30.61)
  line L466 (-9.1, -30.61) -> (-9.1, -29.61)
  line L467 (-9.1, -29.61) -> (-8.1, -29.61)
  line L468 (-8.1, -32.24) -> (-8.1, -33.24)
  line L469 (-8.1, -33.24) -> (-9.1, -33.24)
  line L470 (-9.1, -33.24) -> (-9.1, -32.24)
  line L471 (-9.1, -32.24) -> (-8.1, -32.24)
  line L472 (-8.1, -34.87) -> (-8.1, -35.87)
  line L473 (-8.1, -35.87) -> (-9.1, -35.87)
  line L474 (-9.1, -35.87) -> (-9.1, -34.87)
  line L475 (-9.1, -34.87) -> (-8.1, -34.87)
  line L476 (-8.1, -37.5) -> (-8.1, -38.5)
  line L477 (-8.1, -38.5) -> (-9.1, -38.5)
  line L478 (-9.1, -38.5) -> (-9.1, -37.5)
  line L479 (-9.1, -37.5) -> (-8.1, -37.5)
  line L480 (-5.3, 38.77) -> (-5.3, 37.77)
  line L481 (-5.3, 37.77) -> (-6.3, 37.77)
  line L482 (-6.3, 37.77) -> (-6.3, 38.77)
  line L483 (-6.3, 38.77) -> (-5.3, 38.77)
  line L484 (-5.3, 36.14) -> (-5.3, 35.14)
  line L485 (-5.3, 35.14) -> (-6.3, 35.14)
  line L486 (-6.3, 35.14) -> (-6.3, 36.14)
  line L487 (-6.3, 36.14) -> (-5.3, 36.14)
  line L488 (-5.3, 33.51) -> (-5.3, 32.51)
  line L489 (-5.3, 32.51) -> (-6.3, 32.51)
  line L490 (-6.3, 32.51) -> (-6.3, 33.51)
  line L491 (-6.3, 33.51) -> (-5.3, 33.51)
  line L492 (-5.3, 30.88) -> (-5.3, 29.88)
  line L493 (-5.3, 29.88) -> (-6.3, 29.88)
  line L494 (-6.3, 29.88) -> (-6.3, 30.88)
  line L495 (-6.3, 30.88) -> (-5.3, 30.88)
  line L496 (-5.3, 28.25) -> (-5.3, 27.25)
  line L497 (-5.3, 27.25) -> (-6.3, 27.25)
  line L498 (-6.3, 27.25) -> (-6.3, 28.25)
  line L499 (-6.3, 28.25) -> (-5.3, 28.25)
  line L500 (-5.3, 25.62) -> (-5.3, 24.62)
  line L501 (-5.3, 24.62) -> (-6.3, 24.62)
  line L502 (-6.3, 24.62) -> (-6.3, 25.62)
  line L503 (-6.3, 25.62) -> (-5.3, 25.62)
  line L504 (-5.3, 22.99) -> (-5.3, 21.99)
  line L505 (-5.3, 21.99) -> (-6.3, 21.99)
  line L506 (-6.3, 21.99) -> (-6.3, 22.99)
  line L507 (-6.3, 22.99) -> (-5.3, 22.99)
  line L508 (-5.3, 20.36) -> (-5.3, 19.36)
  line L509 (-5.3, 19.36) -> (-6.3, 19.36)
  line L510 (-6.3, 19.36) -> (-6.3, 20.36)
  line L511 (-6.3, 20.36) -> (-5.3, 20.36)
  line L512 (-5.3, 17.73) -> (-5.3, 16.73)
  line L513 (-5.3, 16.73) -> (-6.3, 16.73)
  line L514 (-6.3, 16.73) -> (-6.3, 17.73)
  line L515 (-6.3, 17.73) -> (-5.3, 17.73)
  line L516 (-5.3, 15.1) -> (-5.3, 14.1)
  line L517 (-5.3, 14.1) -> (-6.3, 14.1)
  line L518 (-6.3, 14.1) -> (-6.3, 15.1)
  line L519 (-6.3, 15.1) -> (-5.3, 15.1)
  line L520 (-5.3, 12.47) -> (-5.3, 11.47)
  line L521 (-5.3, 11.47) -> (-6.3, 11.47)
  line L522 (-6.3, 11.47) -> (-6.3, 12.47)
  line L523 (-6.3, 12.47) -> (-5.3, 12.47)
  line L524 (-5.3, 9.84) -> (-5.3, 8.84)
  line L525 (-5.3, 8.84) -> (-6.3, 8.84)
  line L526 (-6.3, 8.84) -> (-6.3, 9.84)
  line L527 (-6.3, 9.84) -> (-5.3, 9.84)
  line L528 (-5.3, 7.21) -> (-5.3, 6.21)
  line L529 (-5.3, 6.21) -> (-6.3, 6.21)
  line L530 (-6.3, 6.21) -> (-6.3, 7.21)
  line L531 (-6.3, 7.21) -> (-5.3, 7.21)
  line L532 (-5.3, 4.58) -> (-5.3, 3.58)
  line L533 (-5.3, 3.58) -> (-6.3, 3.58)
  line L534 (-6.3, 3.58) -> (-6.3, 4.58)
  line L535 (-6.3, 4.58) -> (-5.3, 4.58)
  line L536 (-5.3, 1.95) -> (-5.3, 0.95)
  line L537 (-5.3, 0.95) -> (-6.3, 0.95)
  line L538 (-6.3, 0.95) -> (-6.3, 1.95)
  line L539 (-6.3, 1.95) -> (-5.3, 1.95)
  line L540 (-5.3, -0.68) -> (-5.3, -1.68)
  line L541 (-5.3, -1.68) -> (-6.3, -1.68)
  line L542 (-6.3, -1.68) -> (-6.3, -0.68)
  line L543 (-6.3, -0.68) -> (-5.3, -0.68)
  line L544 (-5.3, -3.31) -> (-5.3, -4.31)
  line L545 (-5.3, -4.31) -> (-6.3, -4.31)
  line L546 (-6.3, -4.31) -> (-6.3, -3.31)
  line L547 (-6.3, -3.31) -> (-5.3, -3.31)
  line L548 (-5.3, -5.94) -> (-5.3, -6.94)
  line L549 (-5.3, -6.94) -> (-6.3, -6.94)
  line L550 (-6.3, -6.94) -> (-6.3, -5.94)
  line L551 (-6.3, -5.94) -> (-5.3, -5.94)
  line L552 (-5.3, -8.57) -> (-5.3, -9.57)
  line L553 (-5.3, -9.57) -> (-6.3, -9.57)
  line L554 (-6.3, -9.57) -> (-6.3, -8.57)
  line L555 (-6.3, -8.57) -> (-5.3, -8.57)
  line L556 (-5.3, -11.2) -> (-5.3, -12.2)
  line L557 (-5.3, -12.2) -> (-6.3, -12.2)
  line L558 (-6.3, -12.2) -> (-6.3, -11.2)
  line L559 (-6.3, -11.2) -> (-5.3, -11.2)
  line L560 (-5.3, -13.83) -> (-5.3, -14.83)
  line L561 (-5.3, -14.83) -> (-6.3, -14.83)
  line L562 (-6.3, -14.83) -> (-6.3, -13.83)
  line L563 (-6.3, -13.83) -> (-5.3, -13.83)
  line L564 (-5.3, -16.46) -> (-5.3, -17.46)
  line L565 (-5.3, -17.46) -> (-6.3, -17.46)
  line L566 (-6.3, -17.46) -> (-6.3, -16.46)
  line L567 (-6.3, -16.46) -> (-5.3, -16.46)
  line L568 (-5.3, -19.09) -> (-5.3, -20.09)
  line L569 (-5.3, -20.09) -> (-6.3, -20.09)
  line L570 (-6.3, -20.09) -> (-6.3, -19.09)
  line L571 (-6.3, -19.09) -> (-5.3, -19.09)
  line L572 (-5.3, -21.72) -> (-5.3, -22.72)
  line L573 (-5.3, -22.72) -> (-6.3, -22.72)
  line L574 (-6.3, -22.72) -> (-6.3, -21.72)
  line L575 (-6.3, -21.72) -> (-5.3, -21.72)
  line L576 (-5.3, -24.35) -> (-5.3, -25.35)
  line L577 (-5.3, -25.35) -> (-6.3, -25.35)
  line L578 (-6.3, -25.35) -> (-6.3, -24.35)
  line L579 (-6.3, -24.35) -> (-5.3, -24.35)
  line L580 (-5.3, -26.98) -> (-5.3, -27.98)
  line L581 (-5.3, -27.98) -> (-6.3, -27.98)
  line L582 (-6.3, -27.98) -> (-6.3, -26.98)
  line L583 (-6.3, -26.98) -> (-5.3, -26.98)
  line L584 (-5.3, -29.61) -> (-5.3, -30.61)
  line L585 (-5.3, -30.61) -> (-6.3, -30.61)
  line L586 (-6.3, -30.61) -> (-6.3, -29.61)
  line L587 (-6.3, -29.61) -> (-5.3, -29.61)
  line L588 (-5.3, -32.24) -> (-5.3, -33.24)
  line L589 (-5.3, -33.24) -> (-6.3, -33.24)
  line L590 (-6.3, -33.24) -> (-6.3, -32.24)
  line L591 (-6.3, -32.24) -> (-5.3, -32.24)
  line L592 (-5.3, -34.87) -> (-5.3, -35.87)
  line L593 (-5.3, -35.87) -> (-6.3, -35.87)
  line L594 (-6.3, -35.87) -> (-6.3, -34.87)
  line L595 (-6.3, -34.87) -> (-5.3, -34.87)
  line L596 (-5.3, -37.5) -> (-5.3, -38.5)
  line L597 (-5.3, -38.5) -> (-6.3, -38.5)
  line L598 (-6.3, -38.5) -> (-6.3, -37.5)
  line L599 (-6.3, -37.5) -> (-5.3, -37.5)
  line L600 (-2.5, 38.77) -> (-2.5, 37.77)
  line L601 (-2.5, 37.77) -> (-3.5, 37.77)
  line L602 (-3.5, 37.77) -> (-3.5, 38.77)
  line L603 (-3.5, 38.77) -> (-2.5, 38.77)
  line L604 (-2.5, 36.14) -> (-2.5, 35.14)
  line L605 (-2.5, 35.14) -> (-3.5, 35.14)
  line L606 (-3.5, 35.14) -> (-3.5, 36.14)
  line L607 (-3.5, 36.14) -> (-2.5, 36.14)
  line L608 (-2.5, 33.51) -> (-2.5, 32.51)
  line L609 (-2.5, 32.51) -> (-3.5, 32.51)
  line L610 (-3.5, 32.51) -> (-3.5, 33.51)
  line L611 (-3.5, 33.51) -> (-2.5, 33.51)
  line L612 (-2.5, 30.88) -> (-2.5, 29.88)
  line L613 (-2.5, 29.88) -> (-3.5, 29.88)
  line L614 (-3.5, 29.88) -> (-3.5, 30.88)
  line L615 (-3.5, 30.88) -> (-2.5, 30.88)
  line L616 (-2.5, 28.25) -> (-2.5, 27.25)
  line L617 (-2.5, 27.25) -> (-3.5, 27.25)
  line L618 (-3.5, 27.25) -> (-3.5, 28.25)
  line L619 (-3.5, 28.25) -> (-2.5, 28.25)
  line L620 (-2.5, 25.62) -> (-2.5, 24.62)
  line L621 (-2.5, 24.62) -> (-3.5, 24.62)
  line L622 (-3.5, 24.62) -> (-3.5, 25.62)
  line L623 (-3.5, 25.62) -> (-2.5, 25.62)
  line L624 (-2.5, 22.99) -> (-2.5, 21.99)
  line L625 (-2.5, 21.99) -> (-3.5, 21.99)
  line L626 (-3.5, 21.99) -> (-3.5, 22.99)
  line L627 (-3.5, 22.99) -> (-2.5, 22.99)
  line L628 (-2.5, 20.36) -> (-2.5, 19.36)
  line L629 (-2.5, 19.36) -> (-3.5, 19.36)
  line L630 (-3.5, 19.36) -> (-3.5, 20.36)
  line L631 (-3.5, 20.36) -> (-2.5, 20.36)
  line L632 (-2.5, 17.73) -> (-2.5, 16.73)
  line L633 (-2.5, 16.73) -> (-3.5, 16.73)
  line L634 (-3.5, 16.73) -> (-3.5, 17.73)
  line L635 (-3.5, 17.73) -> (-2.5, 17.73)
  line L636 (-2.5, 15.1) -> (-2.5, 14.1)
  line L637 (-2.5, 14.1) -> (-3.5, 14.1)
  line L638 (-3.5, 14.1) -> (-3.5, 15.1)
  line L639 (-3.5, 15.1) -> (-2.5, 15.1)
  line L640 (-2.5, 12.47) -> (-2.5, 11.47)
  line L641 (-2.5, 11.47) -> (-3.5, 11.47)
  line L642 (-3.5, 11.47) -> (-3.5, 12.47)
  line L643 (-3.5, 12.47) -> (-2.5, 12.47)
  line L644 (-2.5, 9.84) -> (-2.5, 8.84)
  line L645 (-2.5, 8.84) -> (-3.5, 8.84)
  line L646 (-3.5, 8.84) -> (-3.5, 9.84)
  line L647 (-3.5, 9.84) -> (-2.5, 9.84)
  line L648 (-2.5, 7.21) -> (-2.5, 6.21)
  line L649 (-2.5, 6.21) -> (-3.5, 6.21)
  line L650 (-3.5, 6.21) -> (-3.5, 7.21)
  line L651 (-3.5, 7.21) -> (-2.5, 7.21)
  line L652 (-2.5, 4.58) -> (-2.5, 3.58)
  line L653 (-2.5, 3.58) -> (-3.5, 3.58)
  line L654 (-3.5, 3.58) -> (-3.5, 4.58)
  line L655 (-3.5, 4.58) -> (-2.5, 4.58)
  line L656 (-2.5, 1.95) -> (-2.5, 0.95)
  line L657 (-2.5, 0.95) -> (-3.5, 0.95)
  line L658 (-3.5, 0.95) -> (-3.5, 1.95)
  line L659 (-3.5, 1.95) -> (-2.5, 1.95)
  line L660 (-2.5, -0.68) -> (-2.5, -1.68)
  line L661 (-2.5, -1.68) -> (-3.5, -1.68)
  line L662 (-3.5, -1.68) -> (-3.5, -0.68)
  line L663 (-3.5, -0.68) -> (-2.5, -0.68)
  line L664 (-2.5, -3.31) -> (-2.5, -4.31)
  line L665 (-2.5, -4.31) -> (-3.5, -4.31)
  line L666 (-3.5, -4.31) -> (-3.5, -3.31)
  line L667 (-3.5, -3.31) -> (-2.5, -3.31)
  line L668 (-2.5, -5.94) -> (-2.5, -6.94)
  line L669 (-2.5, -6.94) -> (-3.5, -6.94)
  line L670 (-3.5, -6.94) -> (-3.5, -5.94)
  line L671 (-3.5, -5.94) -> (-2.5, -5.94)
  line L672 (-2.5, -8.57) -> (-2.5, -9.57)
  line L673 (-2.5, -9.57) -> (-3.5, -9.57)
  line L674 (-3.5, -9.57) -> (-3.5, -8.57)
  line L675 (-3.5, -8.57) -> (-2.5, -8.57)
  line L676 (-2.5, -11.2) -> (-2.5, -12.2)
  line L677 (-2.5, -12.2) -> (-3.5, -12.2)
  line L678 (-3.5, -12.2) -> (-3.5, -11.2)
  line L679 (-3.5, -11.2) -> (-2.5, -11.2)
  line L680 (-2.5, -13.83) -> (-2.5, -14.83)
  line L681 (-2.5, -14.83) -> (-3.5, -14.83)
  line L682 (-3.5, -14.83) -> (-3.5, -13.83)
  line L683 (-3.5, -13.83) -> (-2.5, -13.83)
  line L684 (-2.5, -16.46) -> (-2.5, -17.46)
  line L685 (-2.5, -17.46) -> (-3.5, -17.46)
  line L686 (-3.5, -17.46) -> (-3.5, -16.46)
  line L687 (-3.5, -16.46) -> (-2.5, -16.46)
  line L688 (-2.5, -19.09) -> (-2.5, -20.09)
  line L689 (-2.5, -20.09) -> (-3.5, -20.09)
  line L690 (-3.5, -20.09) -> (-3.5, -19.09)
  line L691 (-3.5, -19.09) -> (-2.5, -19.09)
  line L692 (-2.5, -21.72) -> (-2.5, -22.72)
  line L693 (-2.5, -22.72) -> (-3.5, -22.72)
  line L694 (-3.5, -22.72) -> (-3.5, -21.72)
  line L695 (-3.5, -21.72) -> (-2.5, -21.72)
  line L696 (-2.5, -24.35) -> (-2.5, -25.35)
  line L697 (-2.5, -25.35) -> (-3.5, -25.35)
  line L698 (-3.5, -25.35) -> (-3.5, -24.35)
  line L699 (-3.5, -24.35) -> (-2.5, -24.35)
  line L700 (-2.5, -26.98) -> (-2.5, -27.98)
  line L701 (-2.5, -27.98) -> (-3.5, -27.98)
  line L702 (-3.5, -27.98) -> (-3.5, -26.98)
  line L703 (-3.5, -26.98) -> (-2.5, -26.98)
  line L704 (-2.5, -29.61) -> (-2.5, -30.61)
  line L705 (-2.5, -30.61) -> (-3.5, -30.61)
  line L706 (-3.5, -30.61) -> (-3.5, -29.61)
  line L707 (-3.5, -29.61) -> (-2.5, -29.61)
  line L708 (-2.5, -32.24) -> (-2.5, -33.24)
  line L709 (-2.5, -33.24) -> (-3.5, -33.24)
  line L710 (-3.5, -33.24) -> (-3.5, -32.24)
  line L711 (-3.5, -32.24) -> (-2.5, -32.24)
  line L712 (-2.5, -34.87) -> (-2.5, -35.87)
  line L713 (-2.5, -35.87) -> (-3.5, -35.87)
  line L714 (-3.5, -35.87) -> (-3.5, -34.87)
  line L715 (-3.5, -34.87) -> (-2.5, -34.87)
  line L716 (-2.5, -37.5) -> (-2.5, -38.5)
  line L717 (-2.5, -38.5) -> (-3.5, -38.5)
  line L718 (-3.5, -38.5) -> (-3.5, -37.5)
  line L719 (-3.5, -37.5) -> (-2.5, -37.5)
  line L720 (-1, -40.5) -> (-1, 40.5)
  line L721 (-1, 40.5) -> (-26.5, 40.5)
  line L722 (-26.5, 40.5) -> (-26.5, -40.5)
  line L723 (-26.5, -40.5) -> (-1, -40.5)
  line L724 (-24, 10.16) -> (-23, 10.16)
  line L725 (-23, 10.16) -> (-23, 9.16)
  line L726 (-23, 9.16) -> (-24, 9.16)
  line L727 (-24, 9.16) -> (-24, 10.16)
  line L728 (-24, 10.16) -> (-23, 9.16) construction
  line L729 (-23, 10.16) -> (-24, 9.16) construction
  line L730 (-26.5, -40.5) -> (-26.5, 40.5)
  point P0 (-23.5, 9.66)
  dimension "d197" = 1
  dimension "d198" = 1
  dimension "d199" = 2.5
  dimension "d200" = 3.7
  constraint horizontal L724
  constraint perpendicular L724 L725
  constraint parallel L724 L726
  constraint parallel L725 L727
  constraint coincident L728 P0
  constraint coincident L729 P0
  measures "d197" distance of L724.start L726.end
  measures "d198" distance of L725.end L726.end
  measures "d199" distance of L727 L730
  measures "d200" distance of L7 L726
extrude "Extrude32" cut sketch "Sketch32" against normal blind 1 contours L724 L725 L726 L727 bodies 1
pattern_linear "R-Pattern10" count 2 spacing 3 along (-1, 0, 0) count 5 spacing 2.63 along (0, -1, 0) of "Extrude32"